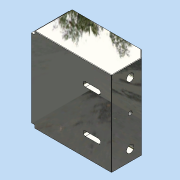
# Autodesk Inventor part: BC-10009
Saved by Autodesk Inventor 2016 (Build 200138000, 138)
## iProperties
Created: 2015-11-25
Part Number: BC-10009
Project: DIPOLO BC-3T- SIRIUS
Cost Center: 1504002005
Material: Aço Carbono AISI 1006
Document SubType Name: Modeling
Designer: reinaldo.basilio
Mass: 35598.3 g
Surface Area: 2271.8 cm^2
Volume: 4523.3 cm^3
Density: 7.87 g/cm^3
Appearance: Silver
Description: Compensador móvel do campo magnético.
RuleStatus: InUse
AfterMaterialChange0: file://_iMaterial
AfterAnyiPropertyChange0: file://_iMaterial
AfterDocNew0: file://_Naming_par
AfterDocNew1: file://_NameStart
AfterDocNew2: file://_NameStart1
AfterDocNew3: file://_Materiais
DocNumber: XXXXX-XXX-XXXX-00-001.ipt
Folder: .
Title: DIPOLO BC-3T- SIRIUS
Author: reinaldo.basilio
Subject: BC-10009
Autodesk Inventor part; units mm, degrees
ref_plane "YZ Plane" through (0, 0, 0) normal (1, 0, 0) x (0, 1, 0)
ref_plane "XZ Plane" through (0, 0, 0) normal (0, 1, 0) x (-1, 0, 0)
ref_plane "XY Plane" through (0, 0, 0) normal (0, 0, 1) x (1, 0, 0)
sketch "Sketch5" plane through (0, 0, 0) normal (0, 1, 0) x (-1, 0, 0)
  line L0 (50, 113) -> (-50, 113)
  line L1 (-50, 113) -> (-50, -113)
  line L2 (-50, -113) -> (50, -113)
  line L3 (50, -113) -> (50, 113)
  point P0 (0, 0)
  point P1 (50, 0)
  point P2 (0, 113)
  dimension "d8" = 100
  dimension "d9" = 226
  constraints: 8 end point, 2 midpoint, 2 parallel, 1 horizontal, 1 horizontal alignment, 1 perpendicular, 1 vertical alignment
  measures "d8" distance of L0.start L0.end
  measures "d9" distance of L0.end L1.end
extrude "Extrusion5" add sketch "Sketch5" along normal blind 215
sketch "Sketch9" plane through (-50, 0, -113) normal (-1, 0, 0) x (0, 0, 1)
  line L0 (0, 215) -> (226, 215) projected
  line L1 (170, 180.25) -> (170, 145.25) construction
  line L2 (163.75, 180.25) -> (163.75, 145.25)
  line L3 (176.25, 145.25) -> (176.25, 180.25)
  arc A0 (176.25, 180.25) -> (163.75, 180.25) centre (170, 180.25) ccw
  arc A1 (163.75, 145.25) -> (176.25, 145.25) centre (170, 145.25) ccw
  line L4 (113, 215) -> (113, 186.8149) construction
  line L5 (56, 180.25) -> (56, 145.25) construction
  line L6 (62.25, 180.25) -> (62.25, 145.25)
  line L7 (49.75, 145.25) -> (49.75, 180.25)
  arc A2 (62.25, 180.25) -> (49.75, 180.25) centre (56, 180.25) ccw
  arc A3 (49.75, 145.25) -> (62.25, 145.25) centre (56, 145.25) ccw
  line L8 (180, 145.25) -> (180, 180.25)
  arc A4 (180, 180.25) -> (160, 180.25) centre (170, 180.25) ccw
  line L9 (160, 180.25) -> (160, 145.25)
  arc A5 (160, 145.25) -> (180, 145.25) centre (170, 145.25) ccw
  line L10 (46, 145.25) -> (46, 180.25)
  arc A6 (66, 180.25) -> (46, 180.25) centre (56, 180.25) ccw
  line L11 (66, 180.25) -> (66, 145.25)
  arc A7 (46, 145.25) -> (66, 145.25) centre (56, 145.25) ccw
  circle A8 centre (170, 145.25) radius 9
  point P0 (113, 0)
  point P1 (170, 162.75)
  point P2 (56, 162.75)
  dimension "d41" = 34.75
  dimension "d42" = 35
  dimension "d44" = 114
  dimension "d45" = 57
  dimension "d46" = 12.5
  dimension "d47" = 20
  dimension "d93" = 18
  constraints: 26 end point, 16 point on circle, 11 symmetric about line, 9 centre point, 4 tangent, 2 midpoint, 2 parallel, 1 coincident, 1 perpendicular, 1 vertical, 7 other
  measures "d41" distance from line of L1.start L0
  measures "d42" distance of L1.start L1.end
  measures "d44" distance between parallel lines of L5 L1
  measures "d45" distance between parallel lines of L4 L1
  measures "d46" distance between parallel lines of L2 L3
  measures "d47" distance between parallel lines of L9 L8
  measures "d93" diameter of A8
extrude "Extrusion7" cut sketch "Sketch9" against normal through all contours A0 L3 A8 L2 | A8 L3 A1 L2 | L6 A3 L7 A2 picked at (169.6717, 148.232)
extrude "Extrusion8" cut sketch "Sketch9" against normal blind 60 contours L2 A1 L3 A8 | A5 L9 A4 L8 | L10 A6 L11 A7 picked at (163.2862, 148.9936)
chamfer "Chamfer4" distance 20 angle 45 1 edges at (-50, 215, 0)
sketch "Sketch10" plane through (0, 215, 0) normal (0, 1, 0) x (1, 0, 0)
  circle A0 centre (0, -82.5) radius 6
  circle A1 centre (0, 82.5) radius 6
  circle A2 centre (0, -82.5) radius 10
  circle A3 centre (0, 82.5) radius 10
  line L0 (50, -113) -> (50, 113) projected
  line L1 (-50, -113) -> (50, -113) projected
  point P0 (0, 0)
  point P1 (0, -113)
  dimension "d55" = 165
  dimension "d56" = 82.5
  dimension "d57" = 12
  dimension "d58" = 20
  dimension "d92" = 50
  constraints: 4 centre point, 2 equal radius, 2 vertical alignment, 1 midpoint
  measures "d55" distance of A1.centre A0.centre
  measures "d56" distance of A0.centre point (0, 0)
  measures "d57" diameter of A0
  measures "d58" diameter of A2
  measures "d92" distance from line of L0 A0.centre
hole "Hole2" at (0, 215, 82.5) at (0, 215, -82.5) direction (0, -1, 0) diameter 20 depth 140
sketch "Sketch11" plane through (0, 75, -82.5) normal (0, 1, 0) x (1, 0, 0)
  circle A0 centre (0, 0) radius 10 projected
  circle A1 centre (0, 0) radius 6
  circle A2 centre (0, -165) radius 6
  circle A3 centre (0, -165) radius 10 projected
  circle A4 centre (0, 0) radius 10 projected
  point P0 (0, -82.5)
  dimension "d66" = 12
  constraints: 2 centre point, 2 concentric, 1 coincident, 1 equal radius
  measures "d66" diameter of A1
hole "Hole3" at (0, 75, -82.5) at (0, 75, 82.5) direction (0, -1, 0) diameter 10.106 end through all thread size "M12x1.75" class "6H" standard "ISO Metric profile"
sketch "Sketch12" plane through (0, 215, 0) normal (0, 1, 0) x (1, 0, 0)
  circle A0 centre (0, -82.5) radius 10 projected
  line L0 (50, -113) -> (50, 113) projected
  circle A1 centre (0, 0) radius 6
  point P0 (50, 0)
  dimension "d74" = 12
  constraints: 1 centre point, 1 horizontal alignment, 1 midpoint, 1 vertical alignment
  measures "d74" diameter of A1
hole "Hole4" at (0, 215, 0) direction (0, -1, 0) diameter 10.106 depth 30 tip angle 118 thread size "M12x1.75" class "6H" standard "ANSI Metric M Profile"
sketch "Sketch13" plane through (-50, 0, -113) normal (-1, 0, 0) x (0, 0, 1)
  line L0 (0, 0) -> (226, 0) projected
  circle A0 centre (113, 107.5) radius 6
  line L1 (0, 0) -> (0, 215) projected
  line L2 (226, 215) -> (0, 215) projected
  point P0 (113, 0)
  point P1 (0, 107.5)
  point P2 (113, 0)
  dimension "d82" = 12
  dimension "d83" = 107.5
  constraints: 2 midpoint, 1 centre point, 1 horizontal alignment, 1 vertical alignment
  measures "d82" diameter of A0
  measures "d83" distance from line of L2 A0.centre
hole "Hole5" at (-50, 107.5, 0) direction (1, 0, 0) diameter 10.106 depth 30 tip angle 118 thread size "M12x1.75" class "6H" standard "ANSI Metric M Profile"
chamfer "Chamfer5" distance 1 angle 45 13 edges at (-50, 97.5, 113) (-40, 205, 113) (10, 215, 113) (10, 215, -113) (-40, 205, -113) (-50, 97.5, -113) (0, 0, -113) (0, 0, 113) (50, 107.5, 113) (50, 107.5, -113) (50, 215, 0) (50, 0, 0) (-50, 0, 0)
sketch "Sketch14" plane through (-50, 1, -112) normal (-1, 0, 0) x (0, 0, 1)
  line L0 (225, -1) -> (216, -1)
  line L1 (216, -1) -> (216, 9)
  line L2 (216, 9) -> (225, 9)
  line L3 (225, 9) -> (225, -1)
  line L4 (225, 0) -> (225, 193.5858) projected
  line L5 (0, -1) -> (224, -1) projected
  line L6 (112, -1) -> (112, -17.0176) construction
  line L7 (-1, -1) -> (8, -1)
  line L8 (8, -1) -> (8, 9)
  line L9 (8, 9) -> (-1, 9)
  line L10 (-1, 9) -> (-1, -1)
  point P0 (-1, 0)
  dimension "d97" = 10
  dimension "d98" = 9
  constraints: 18 end point, 5 symmetric about line, 2 collinear, 2 parallel, 1 horizontal, 1 perpendicular, 1 vertical
  measures "d97" distance of L2.end L0.start
  measures "d98" distance of L1.end L2.end
extrude "Extrusion9" cut sketch "Sketch14" against normal through all
chamfer "Chamfer6" distance 1 angle 45 4 edges at (0, 10, 113) (0, 0, 104) (0, 0, -104) (0, 10, -113)
equation "\"d56\" = 0.5 * d55"
body "Solid5"
